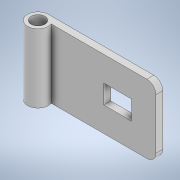
# Autodesk Inventor part: Hinge2
Saved by Autodesk Inventor 2022 (Build 260153000, 153)
## iProperties
Created: 2021-06-15
Part Number: Hinge2
Material: Generic
Document SubType Name: Modeling
Designer: Cornee
Density: 1 g/cm^3
Appearance: Default
Author: Cornee
Autodesk Inventor part; units mm, degrees
ref_plane "YZ Plane" through (0, 0, 0) normal (1, 0, 0) x (0, 1, 0)
ref_plane "XZ Plane" through (0, 0, 0) normal (0, 1, 0) x (-1, 0, 0)
ref_plane "XY Plane" through (0, 0, 0) normal (0, 0, 1) x (1, 0, 0)
sketch "Sketch1" plane through (0, 0, 0) normal (0, 0, 1) x (1, 0, 0)
  line L0 (2.4923, 27.854) -> (38.4923, 27.854)
  line L1 (38.4923, 27.854) -> (38.4923, 8.054)
  line L2 (38.4923, 8.054) -> (2.4923, 8.054)
  line L3 (2.4923, 8.054) -> (2.4923, 27.854)
  line L4 (23.4923, 20.704) -> (31.4923, 20.704)
  line L5 (31.4923, 20.704) -> (31.4923, 15.204)
  line L6 (31.4923, 15.204) -> (23.4923, 15.204)
  line L7 (23.4923, 15.204) -> (23.4923, 20.704)
  point P0 (0, 0)
  dimension "d0" = 36
  dimension "d1" = 19.8
  dimension "d2" = 8
  dimension "d3" = 5.5
  dimension "d4" = 7.15
  dimension "d5" = 7
  constraints: 16 end point, 4 parallel, 2 horizontal, 2 perpendicular
  measures "d0" distance of L1.end L2.end
  measures "d1" distance of L0.end L1.end
  measures "d2" distance of L5.end L6.end
  measures "d3" distance of L4.end L5.end
  measures "d4" distance from line of L0 L4.end
  measures "d5" horizontal distance of L0.end L4.end
extrude "Extrusion1" add sketch "Sketch1" along normal blind 2
fillet "Fillet1" radius 2.6 1 edges at (38.4923, 27.854, 1)
fillet "Fillet2" radius 2.6 1 edges at (38.4923, 8.054, 1)
sketch "Sketch2" plane through (2.4923, 8.054, 0) normal (0, -1, 0) x (1, 0, 0)
  circle A0 centre (3, 3) radius 2
  circle A1 centre (3, 3) radius 3
  line L0 (0, 0) -> (33.4, 0) projected
  line L1 (0, 0) -> (0, 2) projected
  line L2 (33.4, 0) -> (0, 0) projected
  line L3 (3, 0) -> (0, 0)
  line L4 (0, 0) -> (0, 2)
  line L5 (33.4, 2) -> (0, 2) projected
  arc A2 (0.1716, 2) -> (3, 0) centre (3, 3) ccw
  point P0 (-2.4923, 0)
  point P1 (1.2679, 2)
  point P2 (4.7321, 2)
  point P3 (5.8284, 2)
  dimension "d10" = 4
  dimension "d11" = 6
  dimension "d12" = 3
  dimension "d13" = 3
  constraints: 4 end point, 4 point on circle, 3 centre point, 2 coincident, 2 collinear, 2 point on line
  measures "d10" diameter of A0
  measures "d11" diameter of A1
  measures "d12" distance from line of L0 A0.centre
  measures "d13" distance from line of L1 A0.centre
extrude "Extrusion2" cut sketch "Sketch2" against normal through all contours A1 L0 L1 L5
extrude "Extrusion3" add sketch "Sketch2" against normal up to surface (19.8 mm away) contours A0 L5 A1 picked at (5.6161, 3.4074)
extrude "Extrusion4" cut sketch "Sketch2" against normal through all contours L5 A0 picked at (2.772, 1.4585)
body "Solid1"
